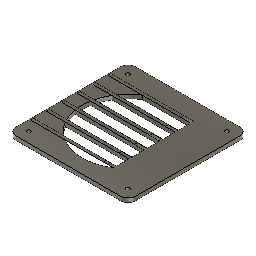
Exhaust pipe external bracket v9 (Autodesk Fusion 360 design; units mm, degrees)
Autodesk Fusion 360 part; units mm, degrees
note: some values were not read from the file. Set by a fixed rule: which sketch regions a step uses.
sketch "Sketch1" plane through (0, 0, 0) normal (0, 0, 1) x (1, 0, 0)
  line L0 (8, 0) -> (118.7, 0)
  line L1 (126.7, 8) -> (126.7, 118.7)
  line L2 (118.7, 126.7) -> (8, 126.7)
  line L3 (0, 118.7) -> (0, 8)
  circle A0 centre (10.85, 10.85) radius 2.15
  circle A1 centre (115.85, 10.85) radius 2.15
  circle A2 centre (10.85, 115.85) radius 2.15
  circle A3 centre (115.85, 115.85) radius 2.15
  arc A4 (8, 126.7) -> (0, 118.7) centre (8, 118.7) ccw
  arc A5 (126.7, 118.7) -> (118.7, 126.7) centre (118.7, 118.7) ccw
  arc A6 (118.7, 0) -> (126.7, 8) centre (118.7, 8) ccw
  arc A7 (0, 8) -> (8, 0) centre (8, 8) ccw
  line L4 (89, 22.1878) -> (89, 104.5122)
  line L5 (89, 104.5122) -> (37.7, 104.5122)
  line L6 (89, 88.1122) -> (21.6477, 88.1122)
  line L7 (89, 71.7122) -> (15.5763, 71.7122)
  line L8 (89, 55.3122) -> (15.5207, 55.3122)
  line L9 (89, 38.9122) -> (21.4567, 38.9122)
  line L10 (89, 22.5122) -> (37.1866, 22.5122)
  line L11 (83.3987, 107.5122) -> (43.3013, 107.5122)
  line L12 (89, 91.1122) -> (23.5818, 91.1122)
  line L13 (89, 74.7122) -> (16.1997, 74.7122)
  line L14 (89, 58.3122) -> (15.5207, 58.3122)
  line L15 (89, 41.9122) -> (21.4567, 41.9122)
  line L16 (89, 25.5122) -> (37.1866, 25.5122)
  line L17 (37.1866, 25.5122) -> (33.0094, 25.5122)
  line L18 (19.8452, 41.9122) -> (21.4567, 41.9122)
  line L19 (15.5207, 58.3122) -> (15.1124, 58.3122)
  arc A8 (89, 104.5122) -> (83.3987, 107.5122) centre (63.35, 63.35) ccw
  arc A9 (43.3013, 107.5122) -> (89, 22.1878) centre (63.35, 63.35) ccw
  point P0 (126.7, 0)
  point P1 (0, 126.7)
  dimension "d1" = 126.7
  dimension "d2" = 126.7
  dimension "d5" = 4.3
  dimension "d6" = 10.85
  dimension "d7" = 10.85
  dimension "d10" = 105
  dimension "d11" = 105
  dimension "d12" = 8
  dimension "d17" = 97
  dimension "d39" = 89
  dimension "d47" = 3
  dimension "d48" = 3
  dimension "d49" = 3
  constraint horizontal L0
  constraint vertical L1
  constraint horizontal L2
  constraint vertical L3
  constraint coincident P1 L2
  constraint coincident P1 L3
  constraint tangent L2 A4
  constraint tangent L3 A4
  constraint tangent L1 A5
  constraint tangent L2 A5
  constraint equal A4 A5
  constraint coincident P0 L0
  constraint coincident P0 L1
  constraint tangent L0 A6
  constraint tangent L1 A6
  constraint equal A4 A6
  constraint coincident origin L0
  constraint coincident origin L3
  constraint tangent L0 A7
  constraint tangent L3 A7
  constraint equal A4 A7
  constraint perpendicular L2 L4
  constraint perpendicular L3 L5
  constraint coincident L5.end A8
  constraint coincident L6.end A8
  constraint coincident L7.end A8
  constraint coincident L8.end A8
  constraint coincident L9.end A8
  constraint coincident L10.end A8
  constraint coincident L17.end A8
  constraint parallel L16 L17
  constraint coincident L18.start A8
  constraint parallel L15 L18
  constraint coincident L19.end A8
  constraint parallel L14 L19
  constraint parallel L5 L11
  constraint coincident L11.end A8
  constraint parallel L6 L12
  constraint coincident L12.end A8
  constraint parallel L7 L13
  constraint coincident L13.end A8
  constraint concentric A8 A9
  measures "d1" distance of origin P0
  measures "d2" distance of origin P1
  measures "d5" diameter of A0
  measures "d6" distance of L0 A0.centre
  measures "d7" distance of L3 A0.centre
  measures "d12" radius of A4
  measures "d17" diameter of A8
  measures "d39" distance of L3 L4
extrude "Extrude1" add sketch "Sketch1" against normal blind 4 makes body 1
ref_plane "WorkPlane5" through (89, 63.35, -2) normal (1, 0, 0) x (0, -1, 0)
sketch "Sketch7" plane through (89, 63.35, -2) normal (1, 0, 0) x (0, 1, 0)
  line L0 (-41, 2) -> (-51.6066, 12.6066)
  line L1 (-41, 2) -> (-31, 2) construction
  line L2 (-38, 2) -> (-48.6066, 12.6066)
  line L3 (-38, 2) -> (-28, 2) construction
  line L4 (-24.6, 2) -> (-35.2066, 12.6066)
  line L5 (-21.6, 2) -> (-32.2066, 12.6066)
  line L6 (-8.2, 2) -> (-18.8066, 12.6066)
  line L7 (-5.2, 2) -> (-15.8066, 12.6066)
  line L8 (8.2, 2) -> (-2.4066, 12.6066)
  line L9 (11.2, 2) -> (0.5934, 12.6066)
  line L10 (24.6, 2) -> (13.9934, 12.6066)
  line L11 (27.6, 2) -> (16.9934, 12.6066)
  line L12 (41, 2) -> (30.3934, 12.6066)
  line L13 (44, 2) -> (33.3934, 12.6066)
  line L14 (-51.6066, 12.6066) -> (-48.6066, 12.6066)
  line L15 (-35.2066, 12.6066) -> (-32.2066, 12.6066)
  line L16 (-18.8066, 12.6066) -> (-15.8066, 12.6066)
  line L17 (-2.4066, 12.6066) -> (0.5934, 12.6066)
  line L18 (13.9934, 12.6066) -> (16.9934, 12.6066)
  line L19 (30.3934, 12.6066) -> (33.3934, 12.6066)
  line L20 (-38, 2) -> (-41, 2)
  line L21 (-21.6, 2) -> (-24.6, 2)
  line L22 (-5.2, 2) -> (-8.2, 2)
  line L23 (11.2, 2) -> (8.2, 2)
  line L24 (27.6, 2) -> (24.6, 2)
  line L25 (44, 2) -> (41, 2)
  dimension "d52" = 135
  dimension "d53" = 15
  dimension "d54" = 135
  dimension "d55" = 15
  dimension "d58" = 16.4
  dimension "d59" = 0
  constraint horizontal L1
  constraint horizontal L3
  constraint coincident L1 L2.start
  measures "d52" angle of L0 L1
  measures "d53" distance of L0.start L0.end
  measures "d54" angle of L2 L3
  measures "d55" distance of L2.start L2.end
extrude "Extrude8" add sketch "Sketch7" against normal blind 77 separate body makes body 2 at (37.6667, 100.8145, 3.5355) makes body 3 at (37.6667, 18.8145, 3.5355) makes body 4 at (63.3333, 84.4145, 3.5355) makes body 5 at (63.3333, 51.6145, 3.5355) makes body 6 at (37.6667, 35.2145, 3.5355) makes body 7 at (63.3333, 68.0145, 3.5355)
extrude "Extrude9" add sketch "Sketch1" against normal blind 4 contours L4 L9 L15 L18 A9 | L4 L8 L14 L19 A9 | L4 L7 L13 A9 | L4 L6 L12 A9 | L5 L11 A8 A9 bodies 1 2 4 5 6 7
combine "Combine1" operation add target body 1 tool bodies 3
equation "d52 = 180 deg - 45 deg"
named bodies: "Exhaust pipe external bracket"
